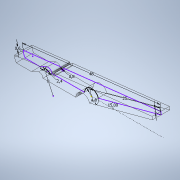
# Autodesk Inventor part: kolik_drivko
Saved by Autodesk Inventor 2022 (Build 260153000, 153)
## iProperties
Created: 2021-05-26
Part Number: kolik_drivko
Material: Všeobecné
Document SubType Name: Modeling
Designer: HP
Density: 1 g/cm^3
Appearance: Výchozí
Author: HP
Autodesk Inventor part; units mm, degrees
ref_plane "YZ Plane" through (0, 0, 0) normal (1, 0, 0) x (0, 1, 0)
ref_plane "XZ Plane" through (0, 0, 0) normal (0, 1, 0) x (-1, 0, 0)
ref_plane "XY Plane" through (0, 0, 0) normal (0, 0, 1) x (1, 0, 0)
sketch "Náčrt1" plane through (0, 0, 0) normal (0, 0, 1) x (1, 0, 0)
  arc A0 (2.3182, 0.6212) -> (-2.4, 0) centre (0, 0) ccw
  line L0 (2.3182, 0.6212) -> (24.1481, 6.4705)
  line L1 (0, 0) -> (25, 0) construction
  line L2 (24.0349, 7.464) -> (24.1481, 6.4705)
  line L3 (-23.6565, 2.0303) -> (-23.5886, 1.4342)
  arc A1 (-13.8, 0) -> (-15.3126, 1.1586) centre (-15, 0) ccw
  arc A2 (-15.3126, 1.1586) -> (-17.8, 0) centre (-13.2286, -6.5652) ccw
  arc A3 (-23.5886, 1.4342) -> (-23.0574, 0) centre (-20.4092, 1.7964) ccw
  line L4 (-23.0574, 0) -> (-17.8, 0)
  line L5 (-13.8, 0) -> (-2.4, 0)
  arc A4 (-10.3974, 2.9371) -> (-9.6026, 3.0277) centre (-10, 2.9824) ccw
  line L6 (-10.3974, 2.9371) -> (-10.4654, 3.5332)
  line L7 (-9.6705, 3.6238) -> (-9.6026, 3.0277)
  line L8 (-23.6565, 2.0303) -> (-10.4654, 3.5332)
  line L9 (-9.6705, 3.6238) -> (24.0349, 7.464)
  dimension "d0" = 4.8
  dimension "d1" = 25
  dimension "d2" = 15
  dimension "d3" = 48
  dimension "d6" = 1
  dimension "d7" = 0.6
  dimension "d10" = 2.4
  dimension "d13" = 4
  dimension "d14" = 8
  dimension "d16" = 0.8
  constraints: 20 end point, 10 point on circle, 8 perpendicular, 5 centre point, 4 tangent, 3 horizontal, 1 coincident
  measures "d0" diameter of A0
  measures "d1" distance of L1.start L0.end
  measures "d2" angle of L1 L0
  measures "d3" distance of L3.start L2.start
  measures "d6" distance of L0.end L2.start
  measures "d7" distance of L3.end L3.start
  measures "d10" diameter of A1
  measures "d13" distance of L5.start L4.end
  measures "d14" radius of A2
  measures "d16" diameter of A4
extrude "Vysunutí1" add sketch "Náčrt1" along normal mid plane 6
